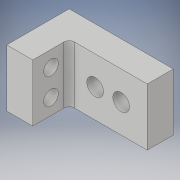
# Autodesk Inventor part: GlyphLiftHolder1
Saved by Autodesk Inventor 2017 (Build 210142000, 142)
## iProperties
Created: 2017-12-29
Part Number: GlyphLiftHolder1
Material: Generic
Document SubType Name: Modeling
Designer: Delta
Density: 1 g/cm^3
Appearance: Default
Author: Delta
Autodesk Inventor part; units mm, degrees
ref_plane "YZ Plane" through (0, 0, 0) normal (1, 0, 0) x (0, 1, 0)
ref_plane "XZ Plane" through (0, 0, 0) normal (0, 1, 0) x (-1, 0, 0)
ref_plane "XY Plane" through (0, 0, 0) normal (0, 0, 1) x (1, 0, 0)
sketch "Sketch1" plane through (0, 0, 0) normal (1, 0, 0) x (0, 1, 0)
  line L0 (0, 0) -> (13.97, 0)
  line L1 (13.97, 0) -> (13.97, -15.24)
  line L2 (13.97, -15.24) -> (0, -15.24)
  line L3 (0, -15.24) -> (0, 0)
  dimension "d0" = 13.97
  dimension "d1" = 15.24
  constraints: 8 end point, 2 parallel, 1 horizontal, 1 perpendicular
  measures "d0" distance of L1.end L2.end
  measures "d1" distance of L0.end L1.end
extrude "Extrusion1" add sketch "Sketch1" along normal blind 6.35
sketch "Sketch2" plane through (6.35, 0, 0) normal (1, 0, 0) x (0, 0, -1)
  line L0 (15.24, 0) -> (15.24, 13.97) projected
  line L1 (0, 0) -> (15.24, 0) projected
  line L2 (15.24, 13.97) -> (8.89, 13.97)
  line L3 (8.89, 13.97) -> (8.89, 0)
  line L4 (8.89, 0) -> (15.24, 0)
  line L5 (15.24, 0) -> (15.24, 13.97)
  dimension "d4" = 6.35
  constraints: 8 end point, 2 parallel, 1 horizontal, 1 perpendicular, 1 point on line
  measures "d4" distance of L4.end L3.end
extrude "Extrusion2" add sketch "Sketch2" along normal blind 19.05
sketch "Sketch3" plane through (6.35, 0, 0) normal (1, 0, 0) x (0, 0, -1)
  line L0 (15.24, 0) -> (0, 0) projected
  line L1 (0, 0) -> (4.445, 0)
  line L2 (4.445, 0) -> (4.445, 3.81)
  line L3 (0, 13.97) -> (15.24, 13.97) projected
  line L4 (4.445, 13.97) -> (4.445, 10.16)
  line L5 (0, 13.97) -> (0, 0) projected
  dimension "d7" = 4.445
  dimension "d8" = 3.81
  dimension "d9" = 3.81
  dimension "d18" = 4.445
  constraints: 6 end point, 2 coincident, 2 point on line, 1 perpendicular, 1 vertical
  measures "d7" distance of L0.end L1.end
  measures "d8" distance of L1.end L2.end
  measures "d9" distance of L4.start L4.end
  measures "d18" distance between parallel lines of L5 L4
hole "Hole1" at (6.35, 10.16, -4.445) at (6.35, 3.81, -4.445) direction (-1, 0, 0) diameter 3.556 depth 25.4 tip angle 118
fillet "Fillet1" radius 1.27 1 edges at (6.35, 6.985, -8.89)
sketch "Sketch4" plane through (25.4, 0, -8.89) normal (0, 0, 1) x (1, 0, 0)
  line L0 (-17.78, 0) -> (0, 0) projected
  line L1 (0, 0) -> (0, 6.985)
  line L2 (0, 13.97) -> (0, 0) projected
  line L3 (0, 6.985) -> (-6.35, 6.985)
  line L4 (-19.05, 13.97) -> (-19.05, 0) projected
  line L5 (-19.05, 6.985) -> (-12.7, 6.985)
  point P0 (-25.4, 0)
  dimension "d19" = 6.35
  dimension "d20" = 6.35
  constraints: 6 end point, 2 coincident, 2 midpoint, 1 horizontal, 1 perpendicular
  measures "d19" distance of L1.end L3.end
  measures "d20" distance of L5.start L5.end
hole "Hole2" at (19.05, 6.985, -8.89) at (12.7, 6.985, -8.89) direction (0, 0, -1) diameter 4.064 depth 25.4 tip angle 118
body "Solid1"
